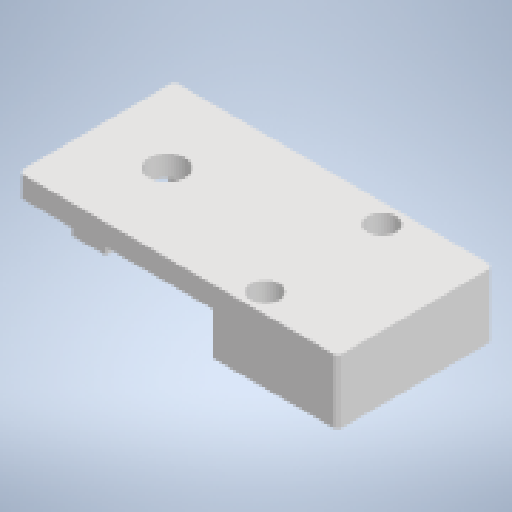
# Autodesk Inventor part: halter_induktivsensor_klein
Saved by Autodesk Inventor 2025 (Build 290162000, 162)
## iProperties
Created: 2025-08-17
Part Number: halter_induktivsensor_klein
Material: Generic
Document SubType Name: Modeling
Designer: peter
Density: 1 g/cm^3
Appearance: Default
Author: peter
Autodesk Inventor part; units mm, degrees
ref_plane "YZ Plane" through (0, 0, 0) normal (1, 0, 0) x (0, 1, 0)
ref_plane "XZ Plane" through (0, 0, 0) normal (0, 1, 0) x (-1, 0, 0)
ref_plane "XY Plane" through (0, 0, 0) normal (0, 0, 1) x (1, 0, 0)
sketch "Sketch1" plane through (0, 0, 0) normal (0, 0, 1) x (1, 0, 0)
  line L0 (13.4, 187.5) -> (13.4, -187.5) projected
  line L1 (0, 187.5) -> (13.4, 187.5) projected
  line L2 (0, 187.5) -> (0, -187.5) projected
  line L3 (13.4, -187.5) -> (0, -187.5) projected
  line L4 (-6.6, 187.5) -> (-6.6, -187.5) projected
  line L5 (-11.3, 187.5) -> (-6.6, 187.5) projected
  line L6 (-11.3, 187.5) -> (-11.3, -187.5) projected
  line L7 (-6.6, -187.5) -> (-11.3, -187.5) projected
  line L8 (24.7, 187.5) -> (24.7, -187.5) projected
  line L9 (20, 187.5) -> (24.7, 187.5) projected
  line L10 (20, 187.5) -> (20, -187.5) projected
  line L11 (24.7, -187.5) -> (20, -187.5) projected
  line L12 (0, -104.7717) -> (51.7, -104.7717)
  line L13 (51.7, -104.7717) -> (51.7, -82.7717)
  line L14 (51.7, -82.7717) -> (0, -82.7717)
  line L15 (0, -82.7717) -> (0, -104.7717)
  line L16 (38.7, -104.7717) -> (38.7, -82.7717) construction
  line L17 (51.7, -93.7717) -> (36.1959, -93.7717) construction
  circle A0 centre (38.7, -101.9917) radius 2
  circle A1 centre (38.7, -85.5517) radius 2
  line L18 (13.4, -93.8117) -> (20, -93.8117) construction
  circle A2 centre (16.7, -93.8117) radius 2.5
  line L19 (6.7, -104.7717) -> (6.7, -82.7717)
  point P0 (0, 0)
  point P1 (0, -82.7717)
  dimension "d0" = 22
  dimension "d3" = 4
  dimension "d4" = 4
  dimension "d5" = 16.44
  dimension "d6" = 14
  dimension "d7" = 5
  dimension "d8" = 27
  constraints: 16 end point, 9 point on line, 4 perpendicular, 3 centre point, 2 horizontal, 2 midpoint, 2 parallel, 1 symmetric about line
  measures "d0" distance between parallel lines of L12 L14
  measures "d3" diameter of A0
  measures "d4" diameter of A1
  measures "d5" distance of A1.centre A0.centre
  measures "d6" distance between parallel lines of L16 L8
  measures "d7" diameter of A2
  measures "d8" distance between parallel lines of L13 L8
extrude "Extrusion1" add sketch "Sketch1" along normal blind 3 contours L14 L10 L12 L0 | L0 L12 L19 L14 | L14 L8 L12 L10 | L14 L13 L12 L8
sketch "Sketch2" plane through (0, 0, 0) normal (0, 0, -1) x (-1, 0, 0)
  line L0 (-14.2, 187.5) -> (-14.2, -187.5) projected
  line L1 (-19.2, 187.5) -> (-19.2, -187.5) projected
  line L2 (-51.7, -82.7717) -> (-6.7, -82.7717) projected
  line L3 (-6.7, -104.7717) -> (-51.7, -104.7717) projected
  line L4 (-51.7, -82.7717) -> (-6.7, -82.7717) projected
  line L5 (-14.3, -82.7717) -> (-19.1, -82.7717)
  line L6 (-19.1, -82.7717) -> (-19.1, -104.7717)
  line L7 (-19.1, -104.7717) -> (-14.3, -104.7717)
  line L8 (-14.3, -104.7717) -> (-14.3, -82.7717)
  circle A0 centre (-16.7, -93.8117) radius 2.5 projected
  line L9 (-19.1, -96.3117) -> (-14.3, -96.3117)
  line L10 (-14.3, -96.3117) -> (-14.3, -91.3117)
  line L11 (-14.3, -91.3117) -> (-19.1, -91.3117)
  line L12 (-19.1, -91.3117) -> (-19.1, -96.3117)
  line L13 (-19.1, -96.3117) -> (-14.3, -91.3117) construction
  line L14 (-14.3, -96.3117) -> (-19.1, -91.3117) construction
  point P0 (0, 0)
  dimension "d9" = 0.1
  dimension "d10" = 0.1
  constraints: 20 end point, 4 parallel, 3 point on line, 2 horizontal, 2 midpoint, 2 perpendicular
  measures "d9" distance between parallel lines of L0 L8
  measures "d10" distance between parallel lines of L1 L6
extrude "Extrusion2" add sketch "Sketch2" along normal blind 1 contours L8 L11 L6 L2 | L3 L6 L9 L8
sketch "Sketch3" plane through (0, 0, 0) normal (0, 0, -1) x (-1, 0, 0)
  line L0 (-51.7, -104.7717) -> (-51.7, -82.7717) projected
  line L1 (-6.7, -104.7717) -> (-51.7, -104.7717) projected
  line L2 (-51.7, -82.7717) -> (-33.7, -82.7717)
  line L3 (-33.7, -82.7717) -> (-33.7, -104.7717)
  line L4 (-33.7, -104.7717) -> (-51.7, -104.7717)
  line L5 (-51.7, -104.7717) -> (-51.7, -82.7717)
  point P0 (0, 0)
  dimension "d13" = 18
  constraints: 8 end point, 2 parallel, 1 horizontal, 1 perpendicular, 1 point on line
  measures "d13" distance of L3.end L4.end
extrude "Extrusion3" add sketch "Sketch3" along normal blind 6
thicken "Thicken1" operation cut thickness 6 both sides no extend neighbours no toward (0, 0, -1) faces at (38.1097, -101.6818, 0)
thicken "Thicken2" operation cut thickness 6 both sides no extend neighbours no toward (0, 0, -1) faces at (38.1097, -85.2418, 0)
chamfer "Chamfer1" distance 0.5 angle 45 6 edges at (33.7, -104.7717, -3) (33.7, -82.7717, -3) (51.7, -104.7717, -1.5) (51.7, -82.7717, -1.5) (6.7, -104.7717, 1.5) (6.7, -82.7717, 1.5)
body "Solid1"
